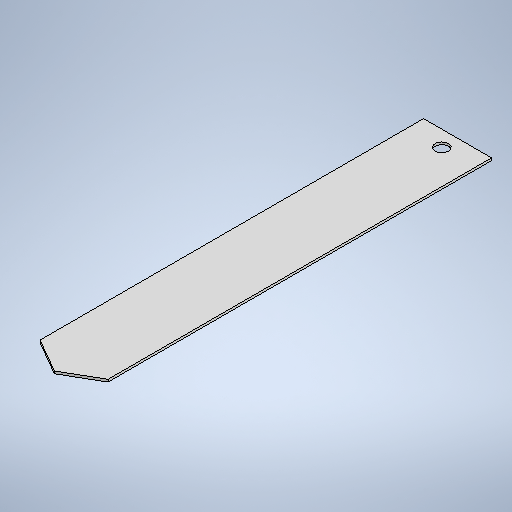
# Autodesk Inventor part: SLM 1696 leg floor pattern
Saved by Autodesk Inventor 2025.3 (Build 293356030, 356C)
## iProperties
Created: 2025-02-20
Part Number: SLM 1696 leg floor pattern
Material: Stainless Steel
Document SubType Name: Sheet Metal
Designer: user
Mass: 1021.57 g
Surface Area: 887.582 cm^2
Volume: 127.696 cm^3
Density: 8 g/cm^3
Sheet Metal Rule: AISI304 3mm Die 32
Sheet Metal Width: 86,000 mm
Sheet Metal Length: 510,000 mm
Sheet Metal Area: 43860,000 mm^2
Appearance: Default
Flat Pattern Width: 8.6 cm
Flat Pattern Length: 51 cm
Flat Pattern Area: 438.6 cm^2
Author: user
Autodesk Inventor part; units mm, degrees
ref_plane "YZ Plane" through (0, 0, 0) normal (1, 0, 0) x (0, 1, 0)
ref_plane "XZ Plane" through (0, 0, 0) normal (0, 1, 0) x (-1, 0, 0)
ref_plane "XY Plane" through (0, 0, 0) normal (0, 0, 1) x (1, 0, 0)
sketch "Sketch6" plane through (0, 0, 0) normal (0, 0, 1) x (1, 0, 0)
  line L0 (0, 0) -> (43, 24.8261)
  line L1 (0, 0) -> (-43, 24.8261)
  line L2 (0, 0) -> (0, 490)
  line L3 (-43, 24.8261) -> (43, 24.8261)
  line L4 (43, 24.8261) -> (43, 510)
  line L5 (43, 510) -> (-43, 510)
  line L6 (-43, 510) -> (-43, 24.8261)
  circle A0 centre (0, 490) radius 8.5
  circle A1 centre (0, 0) radius 490 construction
  circle A2 centre (0, 0) radius 510 construction
  dimension "d44" = 980
  dimension "d40" = 120
  dimension "d42" = 86
  dimension "d43" = 17
  dimension "d45" = 1020
  measures "d40" angle of L0 L1
  measures "d42" distance between parallel lines of L4 L6
  measures "d43" diameter of A0
  measures "d45" diameter of A2
extrude "Plate3" add sketch "Sketch6" along normal blind 3
equation "\"d46\" = Thickness"
equation "\"BendReliefWidth\" = Thickness"
equation "\"BendReliefDepth\" = 0.5 * Thickness"
equation "\"CornerReliefSize\" = 4 * Thickness"
equation "\"MinimumRemnant\" = 2 * Thickness"
equation "\"TransitionRadius\" = BendRadius"
equation "\"JacobiRadiusSize\" = BendRadius"
equation "\"GapSize\" = Thickness"
equation "\"Thickness\" = 3"
equation "\"BendRadius\" = 5"
body "Solid2"
